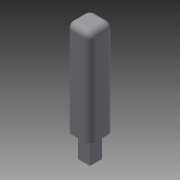
# Autodesk Inventor part: ring1_arm_JacobMorgan_030515_pd3
Saved by Autodesk Inventor 2015 (Build 190159000, 159)
## iProperties
Created: 2015-03-05
Part Number: ring1_arm_JacobMorgan_030515_pd3
Material: Generic
Document SubType Name: Modeling
Designer: WASHHSST
Density: 1 g/cm^3
Appearance: Default
Author: WASHHSST
Autodesk Inventor part; units mm, degrees
ref_plane "YZ Plane" through (0, 0, 0) normal (1, 0, 0) x (0, 1, 0)
ref_plane "XZ Plane" through (0, 0, 0) normal (0, 1, 0) x (-1, 0, 0)
ref_plane "XY Plane" through (0, 0, 0) normal (0, 0, 1) x (1, 0, 0)
sketch "Sketch1" plane through (0, 0, 0) normal (0, 1, 0) x (-1, 0, 0)
  line L0 (0, 0) -> (12.7, 0)
  line L1 (12.7, 0) -> (12.7, -12.7)
  line L2 (12.7, -12.7) -> (0, -12.7)
  line L3 (0, -12.7) -> (0, 0)
  line L4 (0, 0) -> (3.175, 0)
  line L5 (12.7, 0) -> (12.7, -3.175)
  line L6 (12.7, -12.7) -> (12.7, -9.525)
  line L7 (12.7, 0) -> (9.525, 0)
  line L8 (3.175, -3.175) -> (9.525, -3.175)
  line L9 (9.525, -3.175) -> (9.525, -9.525)
  line L10 (9.525, -9.525) -> (3.175, -9.525)
  line L11 (3.175, -9.525) -> (3.175, -3.175)
  dimension "d2" = 12.7
  dimension "d3" = 12.7
  constraints: 24 end point, 4 parallel, 4 point on line, 2 horizontal, 2 perpendicular
  measures "d2" distance of L1.end L2.end
  measures "d3" distance of L0.end L1.end
extrude "Extrusion1" add sketch "Sketch1" along normal blind 12.7 contours L8 L9 L10 L11
sketch "Sketch2" plane through (0, 12.7, 0) normal (0, 1, 0) x (1, 0, 0)
  line L0 (0, 0) -> (-12.7, 0)
  line L1 (-12.7, 0) -> (-12.7, 12.7)
  line L2 (-12.7, 12.7) -> (0, 12.7)
  line L3 (0, 12.7) -> (0, 0)
  dimension "d10" = 12.7
  dimension "d11" = 12.7
  constraints: 8 end point, 2 parallel, 1 horizontal, 1 perpendicular
  measures "d10" distance of L1.end L2.end
  measures "d11" distance of L0.end L1.end
extrude "Extrusion2" add sketch "Sketch2" along normal blind 50.8
fillet "Fillet1" radius 3.175 1 edges at (0, 38.1, 0)
fillet "Fillet2" radius 3.175 1 edges at (0, 38.1, -12.7)
fillet "Fillet3" radius 3.175 1 edges at (-12.7, 38.1, 0)
fillet "Fillet4" radius 3.175 1 edges at (-12.7, 38.1, -12.7)
fillet "Fillet5" radius 3.175 8 edges at (-6.35, 63.5, 0) (-0.9299, 63.5, -0.9299) (0, 63.5, -6.35) (-0.9299, 63.5, -11.7701) (-6.35, 63.5, -12.7) (-11.7701, 63.5, -11.7701) (-12.7, 63.5, -6.35) (-11.7701, 63.5, -0.9299)
body "Solid1"
